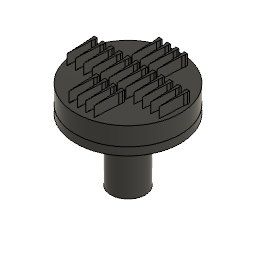
zfish-mold-D20 (Autodesk Fusion 360 design; units mm, degrees)
Autodesk Fusion 360 part; units mm, degrees
sketch "Sketch1" plane through (0, 0, 0) normal (0, 0, 1) x (1, 0, 0)
  line L0 (10, 3.25) -> (-10, 3.25) construction
  line L1 (-10, 3.25) -> (-10, -3.25) construction
  line L2 (-10, -3.25) -> (10, -3.25) construction
  line L3 (10, -3.25) -> (10, 3.25) construction
  line L4 (10, 3.25) -> (-10, -3.25) construction
  line L5 (-10, 3.25) -> (10, -3.25) construction
  line L6 (-9, 2.55) -> (-8.4, 2.55)
  line L7 (-8.4, 2.55) -> (-8.4, 2.15)
  line L8 (-9, 2.15) -> (-9, 2.55)
  line L9 (-8.7, 2.9409) -> (-8.7, -2.4496)
  line L10 (-9, 2.15) -> (-8.9, 1.55)
  line L11 (-8.4, 2.15) -> (-8.5, 1.55)
  line L12 (-8.9, 1.55) -> (-8.7, -2.95)
  line L13 (-8.5, 1.55) -> (-8.7, -2.95)
  line L14 (-7.4, 2.55) -> (-6.8, 2.55)
  line L15 (-7.4, 2.15) -> (-7.4, 2.55)
  line L16 (-7.4, 2.15) -> (-7.3, 1.55)
  line L17 (-7.3, 1.55) -> (-7.1, -2.95)
  line L18 (-6.9, 1.55) -> (-7.1, -2.95)
  line L19 (-6.8, 2.15) -> (-6.9, 1.55)
  line L20 (-6.8, 2.55) -> (-6.8, 2.15)
  line L21 (-5.8, 2.55) -> (-5.2, 2.55)
  line L22 (-5.8, 2.15) -> (-5.8, 2.55)
  line L23 (-5.8, 2.15) -> (-5.7, 1.55)
  line L24 (-5.7, 1.55) -> (-5.5, -2.95)
  line L25 (-5.3, 1.55) -> (-5.5, -2.95)
  line L26 (-5.2, 2.15) -> (-5.3, 1.55)
  line L27 (-5.2, 2.55) -> (-5.2, 2.15)
  line L28 (-4.2, 2.55) -> (-3.6, 2.55)
  line L29 (-4.2, 2.15) -> (-4.2, 2.55)
  line L30 (-4.2, 2.15) -> (-4.1, 1.55)
  line L31 (-4.1, 1.55) -> (-3.9, -2.95)
  line L32 (-3.7, 1.55) -> (-3.9, -2.95)
  line L33 (-3.6, 2.15) -> (-3.7, 1.55)
  line L34 (-3.6, 2.55) -> (-3.6, 2.15)
  line L35 (-2.6, 2.55) -> (-2, 2.55)
  line L36 (-2.6, 2.15) -> (-2.6, 2.55)
  line L37 (-2.6, 2.15) -> (-2.5, 1.55)
  line L38 (-2.5, 1.55) -> (-2.3, -2.95)
  line L39 (-2.1, 1.55) -> (-2.3, -2.95)
  line L40 (-2, 2.15) -> (-2.1, 1.55)
  line L41 (-2, 2.55) -> (-2, 2.15)
  line L42 (-1, 2.55) -> (-0.4, 2.55)
  line L43 (-1, 2.15) -> (-1, 2.55)
  line L44 (-1, 2.15) -> (-0.9, 1.55)
  line L45 (-0.9, 1.55) -> (-0.7, -2.95)
  line L46 (-0.5, 1.55) -> (-0.7, -2.95)
  line L47 (-0.4, 2.15) -> (-0.5, 1.55)
  line L48 (-0.4, 2.55) -> (-0.4, 2.15)
  line L49 (0.6, 2.55) -> (1.2, 2.55)
  line L50 (0.6, 2.15) -> (0.6, 2.55)
  line L51 (0.6, 2.15) -> (0.7, 1.55)
  line L52 (0.7, 1.55) -> (0.9, -2.95)
  line L53 (1.1, 1.55) -> (0.9, -2.95)
  line L54 (1.2, 2.15) -> (1.1, 1.55)
  line L55 (1.2, 2.55) -> (1.2, 2.15)
  circle A0 centre (0, 0) radius 10
  line L56 (2.2, 2.55) -> (2.8, 2.55)
  line L57 (2.2, 2.15) -> (2.2, 2.55)
  line L58 (2.2, 2.15) -> (2.3, 1.55)
  line L59 (2.3, 1.55) -> (2.5, -2.95)
  line L60 (2.7, 1.55) -> (2.5, -2.95)
  line L61 (2.8, 2.15) -> (2.7, 1.55)
  line L62 (2.8, 2.55) -> (2.8, 2.15)
  line L63 (3.8, 2.55) -> (4.4, 2.55)
  line L64 (3.8, 2.15) -> (3.8, 2.55)
  line L65 (3.8, 2.15) -> (3.9, 1.55)
  line L66 (3.9, 1.55) -> (4.1, -2.95)
  line L67 (4.3, 1.55) -> (4.1, -2.95)
  line L68 (4.4, 2.15) -> (4.3, 1.55)
  line L69 (4.4, 2.55) -> (4.4, 2.15)
  line L70 (5.4, 2.55) -> (6, 2.55)
  line L71 (5.4, 2.15) -> (5.4, 2.55)
  line L72 (5.4, 2.15) -> (5.5, 1.55)
  line L73 (5.5, 1.55) -> (5.7, -2.95)
  line L74 (5.9, 1.55) -> (5.7, -2.95)
  line L75 (6, 2.15) -> (5.9, 1.55)
  line L76 (6, 2.55) -> (6, 2.15)
  line L77 (7, 2.55) -> (7.6, 2.55)
  line L78 (7, 2.15) -> (7, 2.55)
  line L79 (7, 2.15) -> (7.1, 1.55)
  line L80 (7.1, 1.55) -> (7.3, -2.95)
  line L81 (7.5, 1.55) -> (7.3, -2.95)
  line L82 (7.6, 2.15) -> (7.5, 1.55)
  line L83 (7.6, 2.55) -> (7.6, 2.15)
  line L84 (8.6, 2.55) -> (9.2, 2.55)
  line L85 (8.6, 2.15) -> (8.6, 2.55)
  line L86 (8.6, 2.15) -> (8.7, 1.55)
  line L87 (8.7, 1.55) -> (8.9, -2.95)
  line L88 (9.1, 1.55) -> (8.9, -2.95)
  line L89 (9.2, 2.15) -> (9.1, 1.55)
  line L90 (9.2, 2.55) -> (9.2, 2.15)
  line L91 (-2.6, 8.55) -> (-2, 8.55)
  line L92 (-2.6, 8.15) -> (-2.6, 8.55)
  line L93 (-2.6, 8.15) -> (-2.5, 7.55)
  line L94 (-2.5, 7.55) -> (-2.3, 3.05)
  line L95 (-2, 8.55) -> (-2, 8.15)
  line L96 (-2, 8.15) -> (-2.1, 7.55)
  line L97 (-2.1, 7.55) -> (-2.3, 3.05)
  line L98 (-1, 8.55) -> (-0.4, 8.55)
  line L99 (-1, 8.15) -> (-1, 8.55)
  line L100 (-1, 8.15) -> (-0.9, 7.55)
  line L101 (-0.9, 7.55) -> (-0.7, 3.05)
  line L102 (-0.5, 7.55) -> (-0.7, 3.05)
  line L103 (-0.4, 8.15) -> (-0.5, 7.55)
  line L104 (-0.4, 8.55) -> (-0.4, 8.15)
  line L105 (0.6, 8.55) -> (1.2, 8.55)
  line L106 (0.6, 8.15) -> (0.6, 8.55)
  line L107 (0.6, 8.15) -> (0.7, 7.55)
  line L108 (0.7, 7.55) -> (0.9, 3.05)
  line L109 (1.1, 7.55) -> (0.9, 3.05)
  line L110 (1.2, 8.15) -> (1.1, 7.55)
  line L111 (1.2, 8.55) -> (1.2, 8.15)
  line L112 (2.2, 8.55) -> (2.8, 8.55)
  line L113 (2.2, 8.15) -> (2.2, 8.55)
  line L114 (2.2, 8.15) -> (2.3, 7.55)
  line L115 (2.3, 7.55) -> (2.5, 3.05)
  line L116 (2.7, 7.55) -> (2.5, 3.05)
  line L117 (2.8, 8.15) -> (2.7, 7.55)
  line L118 (2.8, 8.55) -> (2.8, 8.15)
  line L119 (-2.6, -3.45) -> (-2, -3.45)
  line L120 (-2.6, -3.85) -> (-2.6, -3.45)
  line L121 (-2.6, -3.85) -> (-2.5, -4.45)
  line L122 (-2.5, -4.45) -> (-2.3, -8.95)
  line L123 (-2.1, -4.45) -> (-2.3, -8.95)
  line L124 (-2, -3.85) -> (-2.1, -4.45)
  line L125 (-2, -3.45) -> (-2, -3.85)
  line L126 (-1, -3.45) -> (-0.4, -3.45)
  line L127 (-1, -3.85) -> (-1, -3.45)
  line L128 (-1, -3.85) -> (-0.9, -4.45)
  line L129 (-0.9, -4.45) -> (-0.7, -8.95)
  line L130 (-0.5, -4.45) -> (-0.7, -8.95)
  line L131 (-0.4, -3.85) -> (-0.5, -4.45)
  line L132 (-0.4, -3.45) -> (-0.4, -3.85)
  line L133 (0.6, -3.45) -> (1.2, -3.45)
  line L134 (0.6, -3.85) -> (0.6, -3.45)
  line L135 (0.6, -3.85) -> (0.7, -4.45)
  line L136 (0.7, -4.45) -> (0.9, -8.95)
  line L137 (1.1, -4.45) -> (0.9, -8.95)
  line L138 (1.2, -3.85) -> (1.1, -4.45)
  line L139 (1.2, -3.45) -> (1.2, -3.85)
  line L140 (2.2, -3.45) -> (2.8, -3.45)
  line L141 (2.2, -3.85) -> (2.2, -3.45)
  line L142 (2.2, -3.85) -> (2.3, -4.45)
  line L143 (2.3, -4.45) -> (2.5, -8.95)
  line L144 (2.7, -4.45) -> (2.5, -8.95)
  line L145 (2.8, -3.85) -> (2.7, -4.45)
  line L146 (2.8, -3.45) -> (2.8, -3.85)
  dimension "d1" = 20
  dimension "d2" = 6.5
  dimension "d3" = 0.6
  dimension "d4" = 0.4
  dimension "d5" = 0.7
  dimension "d6" = 1
  dimension "d7" = 0.4
  dimension "d8" = 5.5
  dimension "d9" = 0.6
  dimension "d12" = 1.6
  dimension "d13" = 0
  dimension "d20" = 20
  dimension "d23" = 1.473
  dimension "d24" = 6
  dimension "d27" = 1.6
  dimension "d28" = -12
  constraint horizontal L0
  constraint perpendicular L0 L1
  constraint parallel L0 L2
  constraint parallel L1 L3
  constraint coincident L4 A0.centre
  constraint coincident L5 A0.centre
  constraint coincident A0.centre origin
  constraint horizontal L6
  constraint vertical L7
  constraint vertical L8
  constraint perpendicular L0 L9
  constraint symmetric L7 L8 L9
  constraint horizontal L10.end L11.end
  constraint symmetric L9 L10.end L11.end
  constraint coincident L9 L12.end
  constraint equal L7 L8
  measures "d1" distance of L1.end L2.end
  measures "d2" distance of L0.end L1.end
  measures "d3" distance of L6.start L6.end
  measures "d4" distance of L6.start L8.start
  measures "d5" distance of L0 L6
  measures "d6" distance of L1 L8
  measures "d7" distance of L10.end L11.end
  measures "d8" distance of L6 L12.end
  measures "d9" vertical distance of L7.end L11.end
  measures "d20" diameter of A0
extrude "Extrude3" add sketch "Sketch1" against normal blind 5 contours L6 L7 L8 L10 L11 L12 L13 | L14 L15 L16 L17 L18 L19 L20 | L21 L22 L23 L24 L25 L26 L27 | L28 L29 L30 L31 L32 L33 L34 | L35 L36 L37 L38 L39 L40 L41 | L42 L43 L44 L45 L46 L47 L48 | L49 L50 L51 L52 L53 L54 L55 | A0 | L56 L57 L58 L59 L60 L61 L62 | L63 L64 L65 L66 L67 L68 L69 | L70 L71 L72 L73 L74 L75 L76 | L77 L78 L79 L80 L81 L82 L83 | L84 L85 L86 L87 L88 L89 L90 | L91 L92 L93 L94 L95 L96 L97 | L98 L99 L100 L101 L102 L103 L104 | L105 L106 L107 L108 L109 L110 L111 | L112 L113 L114 L115 L116 L117 L118 | L119 L120 L121 L122 L123 L124 L125 | L126 L127 L128 L129 L130 L131 L132 | L133 L134 L135 L136 L137 L138 L139 | L140 L141 L142 L143 L144 L145 L146 makes body 1
extrude "Extrude1" add sketch "Sketch1" along normal blind 2 contours L6 L7 L8 L10 L11 L12 L13 | L14 L15 L16 L17 L18 L19 L20 | L21 L22 L23 L24 L25 L26 L27 | L28 L29 L30 L31 L32 L33 L34 | L35 L36 L37 L38 L39 L40 L41 | L42 L43 L44 L45 L46 L47 L48 | L49 L50 L51 L52 L53 L54 L55 | L56 L57 L58 L59 L60 L61 L62 | L63 L64 L65 L66 L67 L68 L69 | L70 L71 L72 L73 L74 L75 L76 | L77 L78 L79 L80 L81 L82 L83 | L84 L85 L86 L87 L88 L89 L90 | L91 L92 L93 L94 L95 L96 L97 | L98 L99 L100 L101 L102 L103 L104 | L105 L106 L107 L108 L109 L110 L111 | L112 L113 L114 L115 L116 L117 L118 | L119 L120 L121 L122 L123 L124 L125 | L126 L127 L128 L129 L130 L131 L132 | L133 L134 L135 L136 L137 L138 L139 | L140 L141 L142 L143 L144 L145 L146 bodies 1
sketch "Sketch2" plane through (0, 0, -5) normal (0, 0, -1) x (1, 0, 0)
  circle A0 centre (0, 0) radius 10
  circle A1 centre (0, 0) radius 7.5
  line L0 (6.3443, -4) -> (2.8723, -2)
  line L1 (2.8723, 2) -> (6.3443, 4)
  line L2 (10.7243, 0) -> (-3.1227, 0)
  arc A2 (2.8723, 2) -> (2.8723, -2) centre (0, 0) ccw
  line L3 (6.4487, -3.8294) -> (2.8086, -1.7325)
  arc A3 (2.8086, 1.7325) -> (2.8086, -1.7325) centre (0, 0) ccw
  line L4 (2.8086, 1.7325) -> (6.4487, 3.8294)
  arc A4 (6.0154, -3.5798) -> (6.0154, 3.5798) centre (0, 0) ccw
  line L5 (0, -7.5) -> (0, 7.5)
  line L6 (-6.4487, -3.8294) -> (-2.8086, -1.7325)
  arc A5 (-6.0154, 3.5798) -> (-6.0154, -3.5798) centre (0, 0) ccw
  line L7 (-2.8086, 1.7325) -> (-6.4487, 3.8294)
  line L8 (-6.3443, -4) -> (-2.8723, -2)
  line L9 (-2.8723, 2) -> (-6.3443, 4)
  arc A6 (2.8086, -1.7325) -> (2.8086, 1.7325) centre (0, 0) ccw
  arc A7 (2.8723, -2) -> (2.982, -1.8324) centre (0, 0) ccw
  dimension "d29" = 15
  dimension "d30" = 7
  dimension "d42" = 0.2
  dimension "d43" = 0.5
  dimension "d56" = 8
  dimension "d59" = 4
  constraint coincident A0.centre A1.centre
  constraint coincident A1 L0.start
  constraint coincident A1 L1.end
  constraint horizontal L2
  constraint symmetric L0.end L1.start L2
  constraint symmetric L0.start L1.end L2
  constraint concentric A1 A4
  constraint coincident L3 A4.start
  constraint coincident L4 A4.end
  constraint coincident A1 L5.start
  constraint coincident A1 L5.end
  constraint vertical L5
  constraint symmetric L3.start L5 L6.start
  constraint symmetric L3.end L5 L6.end
  constraint symmetric A3.start L5 L7.start
  constraint symmetric L4.end L5 L7.end
  constraint symmetric A4 L5 A5
  constraint symmetric A4.start L5 A5.end
  constraint symmetric A4.end L5 A5.start
  constraint coincident A0.centre L5
  constraint coincident A1 L6.start
  constraint symmetric L0.start L5 L8.start
  constraint symmetric L0.end L5 L8.end
  constraint symmetric L1.start L5 L9.start
  constraint symmetric L1.end L5 L9.end
  constraint coincident L3.end A3.end
  constraint coincident A3.start L4.start
  constraint coincident L3 A7.end
  constraint coincident A1 L7.end
  measures "d29" diameter of A1
  measures "d30" diameter of A2
  measures "d43" distance of A1 A4
  measures "d56" distance of L0.start L1.end
  measures "d59" distance of L0.end L1.start
extrude "Extrude4" cut sketch "Sketch2" against normal blind 3.5 contours A1 L2 L4 A4 | A1 L2 L3 A4 | A1 L1 A2 A3 L4 L5 | A1 L0 L3 A7 | L2 L3 A4 A6 | L2 L4 A4 A6 | A1 L1 A2 L5 | A1 L0 A2 L5 | L2 A3 L5 A6 | L2 A3 L5 A6 | A1 A2 L5 L9 | A1 A2 L5 L8 | A2 L3 A3 L5 A7 | A3 L5 | A1 A2 L7 L9 | A2 A3 L5 L7 | A1 A2 L6 L8 | A2 A3 L5 L6 | A1 L6 A5 L7 | A2 A3 L6 L7 | A2 L6 A5 L7 bodies 1
extrude "Extrude5" add sketch "Sketch2" against normal blind 1.5 separate body contours A0 | A1 L1 A2 L5 | A1 L0 A2 L5 | A1 A2 L5 L9 | A1 A2 L5 L8 makes body 2
extrude "Extrude8" cut 1 faces at (9.1015, -0.8694, -5) along direction (0, 0, 1) blind 1.5 on bodies 1 bodies 1
extrude "Extrude6" add sketch "Sketch2" along normal blind 1.4 separate body contours L2 L3 A4 A6 | L2 L4 A4 A6 | L2 A3 L5 A6 | L2 A3 L5 A6 | A3 L5 | A2 A3 L6 L7 | A2 L6 A5 L7 makes body 3
extrude "Extrude7" add sketch "Sketch2" along normal blind 15 contours L2 A3 L5 A6 | L2 A3 L5 A6 | A3 L5 bodies 3
fillet "Fillet1" radius 0.5 2 edges at (3.3, 0, -6.4) (-3.3, 0, -6.4) on bodies 3
fillet "Fillet2" radius 0.25 4 edges at (2.8086, -1.7325, -5.95) (-2.8086, -1.7325, -5.95) (2.8086, 1.7325, -5.95) (-2.8086, 1.7325, -5.95) on bodies 3
copy_body "Body->Comp1" bodies 1 removing the originals makes body 4 in component "Stamp"
copy_body "Body->Comp2" bodies 2 removing the originals makes body 5 in component "Stemlock"
copy_body "Body->Comp3" bodies 3 removing the originals makes body 6 in component "Stem"
component "Stamp" placed x (1, 0, 0) y (0, 1, 0) z (0, 0, 1) at (0, 0, 0)
component "Stemlock" placed x (1, 0, 0) y (0, 1, 0) z (0, 0, 1) at (0, 0, 0)
component "Stem" placed x (1, 0, 0) y (0, 1, 0) z (0, 0, 1) at (0, 0, 0)
